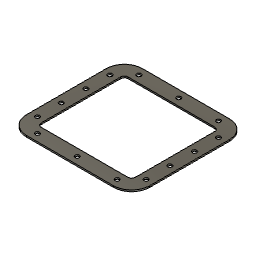
Motor_Mount _Backing_Plate v2 (Autodesk Fusion 360 design; units mm, degrees)
Autodesk Fusion 360 part; units mm, degrees
sketch "Sketch1" plane through (0, 0, 0) normal (0, 0, 1) x (1, 0, 0)
  line L0 (-65, 0) -> (65, 0)
  line L1 (-60, 60) -> (60, 60)
  line L2 (65, 55) -> (65, -55)
  line L3 (60, -60) -> (-60, -60)
  line L4 (-65, -55) -> (-65, 55)
  line L5 (-65, 60) -> (65, -60) construction
  line L6 (65, 60) -> (-65, -60) construction
  line L7 (-65, 0) -> (-85, 0) construction
  circle A0 centre (-75, 0) radius 3
  line L8 (0, 2.5) -> (0, 20) construction
  line L9 (65, 0) -> (85, 0) construction
  circle A1 centre (75, 0) radius 3
  line L10 (0, 60) -> (0, 80) construction
  circle A2 centre (0, 70) radius 3
  line L11 (20, 0) -> (2.5, 0)
  circle A3 centre (0, -70) radius 3
  line L12 (0, -60) -> (0, -80) construction
  circle A4 centre (-75, -50) radius 3
  circle A5 centre (-75, 50) radius 3
  circle A6 centre (75, 50) radius 3
  circle A7 centre (75, -50) radius 3
  circle A8 centre (-55, 70) radius 3
  circle A9 centre (55, 70) radius 3
  circle A10 centre (-55, -70) radius 3
  circle A11 centre (55, -70) radius 3
  line L13 (-85, 55) -> (-85, -55)
  line L14 (85, 55) -> (85, -55)
  line L15 (-60, 80) -> (60, 80)
  line L16 (-60, -80) -> (60, -80)
  circle A12 centre (49.5242, -49.6041) radius 2.5
  circle A13 centre (-0.0023, -49.6041) radius 2.5
  circle A14 centre (-49.5289, -49.6041) radius 2.5
  circle A15 centre (49.5242, 49.6459) radius 2.5
  circle A16 centre (-0.0023, 49.6459) radius 2.5
  circle A17 centre (-49.5289, 49.6459) radius 2.5
  arc A18 (-65, -55) -> (-60, -60) centre (-60, -55) ccw
  arc A19 (-60, 60) -> (-65, 55) centre (-60, 55) ccw
  arc A20 (65, 55) -> (60, 60) centre (60, 55) ccw
  arc A21 (60, -60) -> (65, -55) centre (60, -55) ccw
  line L17 (-75, 0) -> (-75, 17) construction
  line L18 (-75, 0) -> (-75, -17) construction
  circle A22 centre (-75, -17) radius 3
  circle A23 centre (-75, 17) radius 3
  circle A24 centre (75, -17) radius 3
  circle A25 centre (75, 17) radius 3
  line L19 (75, 0) -> (75, 17) construction
  line L20 (75, 0) -> (75, -17) construction
  arc A26 (-85, -55) -> (-60, -80) centre (-60, -55) ccw
  arc A27 (60, -80) -> (85, -55) centre (60, -55) ccw
  arc A28 (85, 55) -> (60, 80) centre (60, 55) ccw
  arc A29 (-60, 80) -> (-85, 55) centre (-60, 55) ccw
  point P0 (-65, 0)
  point P1 (-85, 80)
  point P2 (-85, -80)
  point P3 (85, -80)
  point P4 (85, 80)
  point P5 (-65, -80)
  point P6 (-85, -60)
  point P7 (-65, 80)
  point P8 (-85, 60)
  point P9 (65, 80)
  point P10 (85, 60)
  point P11 (85, -60)
  point P12 (65, -80)
  dimension "d30" = 65
  dimension "d31" = 130
  dimension "d32" = 120
  dimension "d33" = 20
  dimension "d34" = 6
  dimension "d35" = 20
  dimension "d36" = 6
  dimension "d39" = 0
  dimension "d40" = 50
  dimension "d43" = 55
  dimension "d44" = 0
  dimension "d45" = 5
  dimension "d46" = 5
  dimension "d47" = 5
  dimension "d48" = 20
  dimension "d49" = 20
  dimension "d50" = 20
  dimension "d51" = 20
  dimension "d52" = 20
  dimension "d53" = 20
  dimension "d54" = 20
  dimension "d55" = 20
  dimension "d56" = 5
  dimension "d60" = 17
  dimension "d63" = 0
  dimension "d64" = 17
  dimension "d65" = 25
  constraint coincident P0 L0.start
  constraint horizontal L0
  constraint horizontal L1
  constraint perpendicular L1 L2
  constraint parallel L1 L3
  constraint parallel L2 L4
  constraint coincident L5 origin
  constraint coincident L6 origin
  constraint perpendicular L4 L7
  constraint midpoint L7 A0.centre
  constraint symmetric P0 L8 L0.end
  constraint symmetric L7.end L8 L9.end
  constraint symmetric A0 L8 A1
  constraint vertical L10
  constraint midpoint L10 A2.centre
  constraint symmetric L10.start L11 L12.start
  constraint symmetric L10.end L11 L12.end
  constraint symmetric A2 L11 A3
  constraint symmetric L8 A4 A7
  constraint symmetric L8 A5 A6
  constraint symmetric L11 A8 A10
  constraint symmetric L11 A9 A11
  constraint vertical L13
  constraint perpendicular L14 L15
  constraint symmetric L11 P1 P2
  constraint coincident L7.end L13
  constraint coincident L9.end L14
  constraint coincident L10.end L15
  constraint coincident L12.end L16
  constraint coincident P2 L16
  constraint coincident L13 P2
  constraint coincident P1 L15
  constraint coincident L13 P1
  constraint coincident L15 P4
  constraint coincident L14 P4
  constraint coincident L14 P3
  constraint coincident L16 P3
  constraint coincident L6.end L4
  constraint coincident L6.end L3
  constraint tangent L4 A18
  constraint tangent L3 A18
  constraint coincident L1 L10.start
  constraint coincident L5.start L4
  constraint coincident L5.start L1
  constraint tangent L4 A19
  constraint tangent L1 A19
  constraint equal A18 A19
  constraint coincident L6.start L1
  constraint coincident L6.start L2
  constraint tangent L1 A20
  constraint tangent L2 A20
  constraint equal A18 A20
  constraint coincident L5.end L3
  constraint coincident L5.end L2
  constraint tangent L3 A21
  constraint tangent L2 A21
  constraint equal A18 A21
  constraint coincident L13 P6
  constraint coincident L15 P7
  constraint coincident L15 P9
  constraint coincident L14 P10
  constraint coincident L14 P11
  constraint coincident L16 P12
  constraint coincident L16 P5
  constraint coincident L13 P8
  constraint coincident A0.centre L17.start
  constraint perpendicular L7 L17
  constraint symmetric L11 A0.centre L17.start
  constraint symmetric L11 L17.end L18.end
  constraint symmetric L8 A0.centre A1.centre
  constraint symmetric L8 L17.end A25.centre
  constraint symmetric L8 L18.end A24.centre
  constraint symmetric L8 A22 A24
  constraint symmetric L8 A23 A25
  constraint tangent L13 A26
  constraint tangent L16 A26
  constraint tangent L16 A27
  constraint tangent L14 A27
  constraint equal A26 A27
  constraint tangent L15 A28
  constraint tangent L14 A28
  constraint equal A26 A28
  constraint tangent L15 A29
  constraint tangent L13 A29
  constraint equal A26 A29
  constraint parallel L15 L16
  constraint parallel L13 L14
  measures "d30" distance of origin L0.start
  measures "d31" distance of P0 L0.end
  measures "d32" distance of L6.start L5.end
  measures "d33" distance of P0 L7.end
  measures "d34" diameter of A0
  measures "d35" distance of L10.start L10.end
  measures "d36" diameter of A2
  measures "d45" diameter of A13
  measures "d46" diameter of A14
  measures "d47" diameter of A12
  measures "d48" distance of P2 P5
  measures "d49" distance of P2 P6
  measures "d50" distance of P1 P7
  measures "d51" distance of P1 P8
  measures "d52" distance of P4 P9
  measures "d53" distance of P4 P10
  measures "d54" distance of P3 P11
  measures "d55" distance of P3 P12
  measures "d56" radius of A18
  measures "d60" distance of A0.centre L17.end
  measures "d65" radius of A26
extrude "Extrude1" add sketch "Sketch1" along normal blind 2 contours A0 | A1 | L13 L14 L15 L16 A26 A27 A28 A29
equation "d31 = 65 mm + 65 mm"
equation "d49 = d48"
equation "d51 = d50"
equation "d53 = d52"
equation "d55 = d54"
